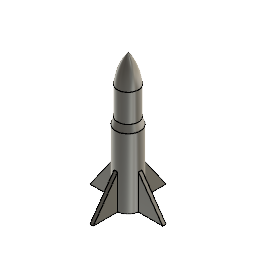
Model Rocket (Autodesk Fusion 360 design; units mm, degrees)
Autodesk Fusion 360 part; units mm, degrees
note: some values were not read from the file. Chosen so that the rebuilt part matches the saved one: which bodies a step acts on; which face or edge a step refers to; where a step ends.
sketch "Sketch1" plane through (0, 0, 0) normal (0, 0, 1) x (1, 0, 0)
  circle A0 centre (0, 0) radius 15
  dimension "d1" = 30
  constraint coincident A0.centre origin
  measures "d1" diameter of A0
extrude "Extrude1" add sketch "Sketch1" along normal blind 150 makes body 1
sketch "Sketch3" plane through (0, 0, 0) normal (1, 0, 0) x (0, 1, 0)
  line L0 (15, 150) -> (-15, 150)
  line L1 (15, 0) -> (-15, 0)
  line L2 (0, 150) -> (-15, 150)
  line L3 (15, 150) -> (0, 150)
  line L4 (0, 0) -> (-15, 0)
  line L5 (15, 0) -> (0, 0)
  line L6 (15, 0) -> (15, 150)
  line L7 (-15, 0) -> (-15, 150)
  line L8 (0, 150) -> (0, 190)
  spline S0 degree 5 poles (0, 190) (0.5101, 189.3429) (1.5118, 188.0159) (2.9584, 185.9875) (4.7736, 183.2057) (6.8406, 179.5912) (8.6886, 175.8278) (10.3012, 171.9043) (11.6722, 167.8166) (12.8142, 163.5732) (13.7457, 159.1867) (14.337, 155.5729) (14.6995, 152.8075) (14.9057, 150.9399) (15, 150) knots 0 0 0 0 0 0 0.1 0.2 0.3 0.4 0.5 0.6 0.7 0.8 0.9 1 1 1 1 1 1
  point P0 (10, 172.5)
  dimension "d5" = 40
  dimension "d6" = 10
  dimension "d7" = 22.5
  constraint coincident L2.start L3.end
  constraint perpendicular L3 L8
  constraint coincident L0.start L3.start
  measures "d5" distance of L2.start L8.end
  measures "d6" distance of L8 P0
  measures "d7" distance of L3 P0
revolve "Revolve1" add sketch "Sketch3" angle 360 about axis through (0, 0, 150) along (0, 0, 1) separate body contours L0 L3 L8 S0 makes body 2
ref_plane "WorkPlane2" through (0, 0, 100) normal (0, 0, -1) x (-1, 0, 0)
split "Split2" by plane through (0, 0, 100) normal (0, 0, -1) bodies 1 makes body 3 at (14.9255, 1.4935, 66.6667)
sketch "Sketch4" plane through (0, 0, 0) normal (0, 0, 1) x (1, 0, 0)
sketch "Sketch5" plane through (0, 0, 0) normal (0, 0, 1) x (1, 0, 0)
sketch "Sketch6" plane through (0, 0, 0) normal (0, 0, 1) x (1, 0, 0)
  circle A0 centre (0, 0) radius 17.5
  dimension "d10" = 35
  constraint coincident A0.centre origin
  measures "d10" diameter of A0
extrude "Extrude2" add sketch "Sketch6" along normal up to surface (100 mm away) bodies 1
sketch "Sketch7" plane through (0, 0, 0) normal (0, 1, 0) x (1, 0, 0)
  line L0 (-17.5, -100) -> (-15, -100)
  line L1 (15, -100) -> (17.5, -100)
  line L2 (-17.5, 0) -> (17.5, 0)
  line L3 (-15, -150) -> (15, -150)
  line L4 (-17.5, 0) -> (-17.5, -100)
  line L5 (17.5, 0) -> (17.5, -100)
  line L6 (-15, -100) -> (-15, -150)
  line L7 (15, -100) -> (15, -150)
  line L8 (15, -110) -> (17.5, -100)
  dimension "d13" = 10
  constraint coincident L7 L8.start
  constraint coincident L1.end L5.end
  measures "d13" distance of L1.start L8.start
revolve "Revolve2" add sketch "Sketch7" angle 360 about axis through (0, 0, 1.75) along (0, 0, 1) separate body contours L1 L7 L8 makes body 4
sketch "Sketch8" plane through (0, 0, 0) normal (0, 1, 0) x (1, 0, 0)
sketch "Sketch9" plane through (0, 0, 0) normal (0, 1, 0) x (1, 0, 0)
sketch "Sketch11" plane through (0, 0, 100) normal (0, 0, -1) x (1, 0, 0)
sketch "Sketch10" plane through (0, 0, 0) normal (1, 0, 0) x (0, 1, 0)
  line L0 (-15, 100) -> (-17.5, 100)
  line L1 (17.5, 100) -> (15, 100)
  line L2 (0, 0) -> (-17.5, 0)
  line L3 (17.5, 0) -> (0, 0)
  line L4 (0, 150) -> (-15, 150)
  line L5 (15, 150) -> (0, 150)
  line L6 (17.5, 0) -> (17.5, 100)
  line L7 (-17.5, 0) -> (-17.5, 100)
  line L8 (15, 100) -> (15, 150)
  line L9 (-15, 100) -> (-15, 150)
  line L10 (17.5, 50) -> (52.5, 0)
  line L11 (52.5, 0) -> (17.5, 0)
  line L12 (17.5, 0) -> (17.5, 50)
  dimension "d15" = 50
  dimension "d16" = 35
  constraint midpoint L6 L10.start
  constraint coincident L3.start L6.start
  constraint perpendicular L6 L11
  measures "d15" distance of L10.start L3.start
  measures "d16" distance of L10.end L3.start
extrude "Extrude3" add sketch "Sketch10" along normal mid plane 5 separate body contours L6 L10 L11 L12 makes body 5
pattern_circular "C-Pattern1" count 4 over 360 about axis through (0, 0, 1.75) along (0, 0, 1) of bodies 5 makes body 6 at (-29.1667, 2.5, 16.6667) makes body 7 at (-2.5, -29.1667, 16.6667) makes body 8 at (29.1667, -2.5, 16.6667)
extrude "Extrude5" add 1 faces at (0.8333, 17.5, 33.3333) along direction (0, -1, 0) up to near side of body 1 on bodies 5 bodies 5 6 7 8 1
extrude "Extrude6" add 1 faces at (17.5, -0.8333, 33.3333) along direction (-1, 0, 0) up to near side of body 5 on bodies 8 bodies 8 6 7 5
extrude "Extrude7" add 1 faces at (-17.5, 0.8333, 33.3333) along direction (1, 0, 0) up to near side of body 8 on bodies 6 bodies 6 8
extrude "Extrude8" add 1 faces at (-0.8333, -17.5, 33.3333) along direction (0, 1, 0) up to near side of body 6 on bodies 7 bodies 7 6
hidden bodies 3
